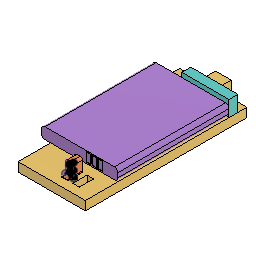
BatteryHolder (Autodesk Fusion 360 design; units mm, degrees)
Autodesk Fusion 360 part; units mm, degrees
sketch "Base" plane through (0, 0, 0) normal (0, 0, 1) x (1, 0, 0) in component "Rail"
  line L0 (0, 0) -> (30, 0)
  line L1 (30, 0) -> (30, 72)
  line L2 (30, 72) -> (0, 72)
  line L3 (0, 72) -> (0, 0)
  line L4 (21, 68) -> (18, 68)
  line L5 (18, 68) -> (18, 28)
  line L6 (18, 28) -> (21, 28)
  line L7 (21, 28) -> (21, 68)
  dimension "d1" = 30
  dimension "d2" = 72
  dimension "d45" = 3
  dimension "d46" = 9
  dimension "d47" = 40
  dimension "d48" = 4
  constraint horizontal L0
  constraint vertical L1
  constraint horizontal L2
  constraint vertical L3
  constraint coincident L0.start L3.end
  constraint horizontal L4
  constraint vertical L5
  constraint horizontal L6
  constraint vertical L7
  measures "d1" distance of L0.start L0.end
  measures "d2" distance of L0.start L2.end
  measures "d45" distance of L4.start L4.end
  measures "d46" distance of L1 L7
  measures "d47" distance of L4.start L6.end
  measures "d48" distance of L2 L4
extrude "Extrude1" add sketch "Base" along normal blind 4 makes body 1 in component "Rail"
sketch "BoltHolder" plane through (0, 0, 4) normal (0, 0, 1) x (-1, 0, 0) in component "Rail"
  line L0 (0, -72) -> (0, 0)
  line L1 (0, 0) -> (-30, 0)
  line L2 (-30, 0) -> (-30, -72)
  line L3 (-30, -72) -> (0, -72)
  line L4 (-23, -72) -> (-16, -72)
  line L5 (-16, -72) -> (-16, -68)
  line L6 (-16, -68) -> (-23, -68)
  line L7 (-23, -68) -> (-23, -72)
  line L8 (-30, 0) -> (-30, -72)
  line L9 (-21, -68) -> (-21, -28)
  line L10 (-21, -28) -> (-18, -28)
  line L11 (-18, -28) -> (-18, -68)
  line L12 (-18, -68) -> (-21, -68)
  dimension "d5" = 7
  dimension "d6" = 4
  dimension "d7" = 7
  constraint horizontal L4
  constraint vertical L5
  constraint horizontal L6
  constraint vertical L7
  constraint coincident L3 L4.start
  measures "d5" distance of L4.start L4.end
  measures "d6" distance of L4.start L6.end
  measures "d7" distance of L7 L8
extrude "Extrude3" add sketch "BoltHolder" along normal blind 7 contours L3 L4 L5 L6 L7 L12 bodies 1 in component "Rail"
sketch "BoltHole" plane through (0, 72, 0) normal (0, 1, 0) x (-1, 0, 0) in component "Rail"
  line L0 (-30, 0) -> (0, 0)
  line L1 (0, 0) -> (0, 4)
  line L2 (0, 4) -> (-16, 4)
  line L3 (-16, 4) -> (-16, 11)
  line L4 (-16, 11) -> (-23, 11)
  line L5 (-23, 11) -> (-23, 4)
  line L6 (-23, 4) -> (-30, 4)
  line L7 (-30, 4) -> (-30, 0)
  line L8 (-23, 11) -> (-16, 4) construction
  line L9 (-23, 4) -> (-16, 11) construction
  circle A0 centre (-19.5, 7.5) radius 1.25
  circle A1 centre (-19.5, 7.5) radius 2.5
  dimension "d12" = 2.5
  dimension "d13" = 5
  constraint coincident L4.end L5.start
  constraint coincident L2.end L3.start
  constraint coincident L5.end L6.start
  constraint coincident L3.end L4.start
  constraint midpoint L8 A0.centre
  constraint concentric A0 A1
  measures "d12" diameter of A0
  measures "d13" diameter of A1
extrude "Extrude4" cut sketch "BoltHole" against normal up to surface (4 mm away) contours A0 bodies 1 in component "Rail"
extrude "Extrude5" cut sketch "BoltHole" against normal blind 2 contours A1 bodies 1 in component "Rail"
sketch "Sketch1" plane through (0, 68, 0) normal (0, -1, 0) x (1, 0, 0) in component "Pusher"
  circle A0 centre (19.5, 7.5) radius 1.25
  line L0 (21, 4) -> (23, 4)
  line L1 (23, 4) -> (23, 11)
  line L2 (23, 11) -> (16, 11)
  line L3 (16, 11) -> (16, 4)
  line L4 (23, 11) -> (30, 11)
  line L5 (30, 11) -> (30, 4)
  line L6 (30, 4) -> (23, 4)
  line L7 (23, 4) -> (23, 11)
  line L8 (16, 11) -> (9, 11)
  line L9 (9, 11) -> (9, 4)
  line L10 (9, 4) -> (16, 4)
  line L11 (16, 4) -> (16, 11)
  line L12 (18, 0) -> (21, 0)
  line L13 (21, 0) -> (21, 4)
  line L14 (16, 4) -> (18, 4)
  line L15 (18, 4) -> (18, 0)
  point P0 (30, 4)
  dimension "d18" = 7
  constraint horizontal L4
  constraint vertical L5
  constraint horizontal L6
  constraint vertical L7
  constraint coincident P0 L5.end
  constraint coincident L1.end L2.start
  constraint horizontal L8
  constraint vertical L9
  constraint horizontal L10
  constraint vertical L11
  constraint coincident L2.end L3.start
  measures "d18" distance of L2.end L8.end
extrude "Extrude1'" add sketch "Sketch1" along normal blind 4 separate body contours A0 | L0 L1 L2 L3 L7 L11 L12 L13 L14 L15 | L1 L4 L5 L6 L7 | L3 L8 L9 L10 L11 makes body 2 in component "Pusher"
sketch "Sketch2" plane through (0, 68, 0) normal (0, 1, 0) x (-1, 0, 0) in component "Pusher"
  line L0 (-9, 11) -> (-30, 11)
  line L1 (-30, 11) -> (-30, 4)
  line L2 (-30, 4) -> (-21, 4)
  line L3 (-9, 4) -> (-9, 11)
  circle A0 centre (-19.5, 7.5) radius 1.25
  line L4 (-21, 4) -> (-21, 0)
  line L5 (-21, 0) -> (-18, 0)
  line L6 (-18, 0) -> (-18, 4)
  line L7 (-18, 4) -> (-9, 4)
extrude "Extrude2" cut sketch "Sketch2" against normal blind 2 contours A0 bodies 2 in component "Pusher"
sketch "Sketch1 (2)" plane through (0, 0, 4) normal (0, 0, 1) x (-1, 0, 0) in component "Connector"
  line L0 (-24.5, -4) -> (-14.5, -4)
  line L1 (-14.5, -4) -> (-14.5, -10)
  line L2 (-14.5, -10) -> (-24.5, -10)
  line L3 (-24.5, -10) -> (-24.5, -4)
  line L4 (0, 0) -> (-30, 0)
  line L5 (-19.5, -72) -> (-19.5, 0) construction
  point P0 (-19.5, -72)
  point P1 (-19.5, -4)
  dimension "d23" = 10
  dimension "d24" = 6
  dimension "d25" = 4
  constraint horizontal L0
  constraint vertical L1
  constraint horizontal L2
  constraint vertical L3
  constraint coincident P0 L5.start
  constraint coincident L4 L5.end
  constraint perpendicular L4 L5
  constraint coincident L5 P1
  constraint midpoint L0 P1
  measures "d23" distance of L0.start L0.end
  measures "d24" distance of L0.start L2.end
  measures "d25" distance of L5.end P1
extrude "Extrude1''" add sketch "Sketch1 (2)" along normal blind 6 separate body makes body 3 in component "Connector"
sketch "Sketch2 (2)" plane through (0, 10, 0) normal (0, 1, 0) x (-1, 0, 0) in component "Connector"
  line L0 (-24.5, 4) -> (-14.5, 4)
  line L1 (-14.5, 4) -> (-14.5, 10)
  line L2 (-14.5, 10) -> (-24.5, 10)
  line L3 (-24.5, 10) -> (-24.5, 4)
  line L4 (-24.5, 10) -> (-14.5, 4) construction
  line L5 (-24.5, 4) -> (-14.5, 10) construction
  circle A0 centre (-19.5, 7) radius 0.75
  dimension "d28" = 1.5
  constraint coincident L2.end L3.start
  constraint coincident L0.end L1.start
  constraint coincident L0.start L3.end
  constraint coincident L1.end L2.start
  constraint midpoint L4 A0.centre
  measures "d28" diameter of A0
extrude "Extrude2'" cut sketch "Sketch2 (2)" against normal up to surface (6 mm away) contours A0 bodies 3 in component "Connector"
pattern_linear "R-Pattern1" count 3 spacing 2.5 along (1, 0, 0) both ways of "Extrude2'" in component "Connector"
sketch "Sketch3" plane through (0, 10, 0) normal (0, 1, 0) x (-1, 0, 0) in component "Connector"
  circle A0 centre (-22, 7) radius 0.75
  line L0 (-24.5, 4) -> (-14.5, 4)
  line L1 (-14.5, 4) -> (-14.5, 10)
  line L2 (-14.5, 10) -> (-24.5, 10)
  line L3 (-24.5, 10) -> (-24.5, 4)
  line L4 (-24.5, 10) -> (-14.5, 4) construction
  line L5 (-24.5, 4) -> (-14.5, 10) construction
  line L6 (-15.3, 5.75) -> (-23.7, 5.75)
  line L7 (-23.7, 5.75) -> (-23.7, 8.25)
  line L8 (-23.7, 8.25) -> (-15.3, 8.25)
  line L9 (-15.3, 8.25) -> (-15.3, 5.75)
  circle A1 centre (-17, 7) radius 0.75
  circle A2 centre (-19.5, 7) radius 0.75
  point P0 (-19.5, 7)
  dimension "d35" = 8.4
  dimension "d36" = 2.5
  constraint coincident L2.end L3.start
  constraint coincident L0.end L1.start
  constraint coincident L0.start L3.end
  constraint coincident L1.end L2.start
  constraint horizontal L6
  constraint perpendicular L6 L7
  constraint parallel L6 L8
  constraint parallel L7 L9
  measures "d35" distance of L7.end L8.end
  measures "d36" distance of L6.end L7.end
extrude "Extrude3'" cut sketch "Sketch3" against normal blind 5.5 contours L6 L7 L8 L9 | A1 | A2 bodies 3 in component "Connector"
sketch "Sketch4" plane through (0, 0, 4) normal (0, 0, -1) x (1, 0, 0) in component "Connector"
  line L0 (14.5, -10) -> (24.5, -10)
  line L1 (24.5, -10) -> (24.5, -4)
  line L2 (24.5, -4) -> (14.5, -4)
  line L3 (14.5, -4) -> (14.5, -10)
  line L4 (19.5, -4) -> (19.5, -10) construction
  line L5 (15.75, -4) -> (18.25, -4)
  line L6 (18.25, -4) -> (18.25, -10)
  line L7 (18.25, -10) -> (15.75, -10)
  line L8 (15.75, -10) -> (15.75, -4)
  line L9 (23.25, -10) -> (23.25, -4)
  line L10 (23.25, -4) -> (20.75, -4)
  line L11 (20.75, -10) -> (23.25, -10)
  line L12 (20.75, -4) -> (20.75, -10)
  line L13 (18.75, -4) -> (20.25, -4)
  line L14 (16.25, -4) -> (17.75, -4)
  point P0 (17, -4)
  dimension "d39" = 2.5
  constraint midpoint L2 L4.start
  constraint midpoint L0 L4.end
  constraint horizontal L5
  constraint vertical L6
  constraint horizontal L7
  constraint vertical L8
  constraint coincident L2 L5.start
  constraint midpoint L5 P0
  constraint symmetric L4 L5.start L9.end
  constraint symmetric L4 L5.end L10.end
  constraint symmetric L4 L6.end L11.start
  constraint symmetric L4 L7.end L9.start
  measures "d39" distance of L5.start L5.end
extrude "Extrude4'" add sketch "Sketch4" along normal blind 4 contours L0 L2 L5 L6 L7 L8 L14 | L0 L2 L9 L10 L11 L12 bodies 3 in component "Connector"
sketch "CutoutConnector" plane through (0, 0, 0) normal (0, 0, 1) x (1, 0, 0) in component "Rail"
  line L0 (15.75, 4) -> (18.25, 4)
  line L1 (18.25, 4) -> (18.25, 10)
  line L2 (18.25, 10) -> (15.75, 10)
  line L3 (15.75, 10) -> (15.75, 4)
  line L4 (20.75, 4) -> (23.25, 4)
  line L5 (23.25, 4) -> (23.25, 10)
  line L6 (23.25, 10) -> (20.75, 10)
  line L7 (20.75, 10) -> (20.75, 4)
  line L8 (18.45, 3.8) -> (18.45, 10.2)
  line L9 (18.45, 10.2) -> (15.55, 10.2)
  line L10 (15.55, 10.2) -> (15.55, 3.8)
  line L11 (15.55, 3.8) -> (18.45, 3.8)
  line L12 (20.55, 10.2) -> (20.55, 3.8)
  line L13 (20.55, 3.8) -> (23.45, 3.8)
  line L14 (23.45, 3.8) -> (23.45, 10.2)
  line L15 (23.45, 10.2) -> (20.55, 10.2)
  point P0 (15.75, 4)
  point P1 (18.25, 10)
  point P2 (20.75, 4)
  point P3 (23.25, 10)
  dimension "d42" = 0.2
  constraint horizontal L0
  constraint vertical L1
  constraint horizontal L2
  constraint vertical L3
  constraint coincident P1 L1.end
  constraint coincident P0 L0.start
  constraint horizontal L4
  constraint vertical L5
  constraint horizontal L6
  constraint vertical L7
  constraint coincident P3 L5.end
  constraint coincident P2 L4.start
extrude "Extrude6" cut sketch "CutoutConnector" along normal up to surface (4 mm away) contours L0 L1 L2 L3 | L4 L5 L6 L7 | L8 L9 L10 L11 | L12 L13 L14 L15 bodies 1 in component "Rail"
sketch "Sketch1 (3)" plane through (0, 0, 4) normal (0, 0, 1) x (-1, 0, 0) in component "WireConnector"
  line L0 (-18.45, -10.2) -> (-18.45, -3.8)
  line L1 (-18.45, -3.8) -> (-15.55, -3.8)
  line L2 (-15.55, -3.8) -> (-15.55, -10.2)
  line L3 (-15.55, -10.2) -> (-18.45, -10.2)
  line L4 (-16, -68) -> (-16, -72)
  line L5 (-16, -72) -> (0, -72)
  line L6 (0, -72) -> (0, 0)
  line L7 (0, 0) -> (-30, 0)
  line L8 (-30, 0) -> (-30, -72)
  line L9 (-30, -72) -> (-23, -72)
  line L10 (-23, -72) -> (-23, -68)
  line L11 (-23, -68) -> (-21, -68)
  line L12 (-21, -68) -> (-21, -28)
  line L13 (-21, -28) -> (-18, -28)
  line L14 (-18, -28) -> (-18, -68)
  line L15 (-18, -68) -> (-16, -68)
  line L16 (-15.55, -10.2) -> (-18.45, -10.2)
  line L17 (-18.45, -10.2) -> (-18.45, -3.8)
  line L18 (-18.45, -3.8) -> (-15.55, -3.8)
  line L19 (-15.55, -3.8) -> (-15.55, -10.2)
  line L20 (-18.25, -10) -> (-18.25, -4)
  line L21 (-18.25, -4) -> (-15.75, -4)
  line L22 (-15.75, -4) -> (-15.75, -10)
  line L23 (-15.75, -10) -> (-18.25, -10)
  constraint horizontal L16
  constraint vertical L17
  constraint horizontal L18
  constraint vertical L19
  constraint coincident L0.end L1.start
  constraint coincident L2.end L3.start
  constraint parallel L17 L20
  constraint parallel L18 L21
  constraint parallel L19 L22
  constraint parallel L16 L23
extrude "Extrude1'''" add sketch "Sketch1 (3)" against normal up to surface (4 mm away) separate body contours L20 L21 L22 L23 makes body 4 in component "WireConnector"
sketch "Sketch2 (3)" plane through (0, 0, 4) normal (0, 0, 1) x (-1, 0, 0) in component "WireConnector"
  line L0 (-15.75, -10) -> (-15.75, -4)
  line L1 (-15.75, -4) -> (-18.25, -4)
  line L2 (-18.25, -4) -> (-18.25, -10)
  line L3 (-18.25, -10) -> (-15.75, -10)
  line L4 (-15.75, -10) -> (-18.25, -10)
  line L5 (-18.25, -10) -> (-18.25, -6)
  line L6 (-18.25, -6) -> (-15.75, -6)
  line L7 (-15.75, -6) -> (-15.75, -10)
  line L8 (-18.25, -10) -> (-18.75, -10)
  line L9 (-18.75, -10) -> (-18.75, -6)
  line L10 (-18.75, -6) -> (-18.25, -6)
  line L11 (-18.25, -6) -> (-18.25, -10)
  line L12 (-15.75, -10) -> (-15.25, -10)
  line L13 (-15.25, -10) -> (-15.25, -6)
  line L14 (-15.25, -6) -> (-15.75, -6)
  line L15 (-15.75, -6) -> (-15.75, -10)
  dimension "d52" = 4
  dimension "d94" = 0.5
  dimension "d95" = 4
  dimension "d96" = 0.5
  constraint horizontal L4
  constraint vertical L5
  constraint horizontal L6
  constraint vertical L7
  constraint coincident L0.start L3.end
  constraint horizontal L8
  constraint vertical L9
  constraint horizontal L10
  constraint vertical L11
  constraint coincident L2.end L3.start
  constraint horizontal L12
  constraint vertical L13
  constraint horizontal L14
  constraint vertical L15
  measures "d52" distance of L0.start L6.end
  measures "d94" distance of L2.end L8.end
  measures "d95" distance of L2.end L5.end
  measures "d96" distance of L0.start L12.end
extrude "Extrude2''" add sketch "Sketch2 (3)" along normal blind 6 contours L0 L2 L3 L4 L5 L6 L7 L11 L15 | L0 L7 L12 L13 L14 L15 | L2 L5 L8 L9 L10 L11 bodies 4 in component "WireConnector"
sketch "Sketch3 (2)" plane through (0, 6, 0) normal (0, -1, 0) x (1, 0, 0) in component "WireConnector"
  line L0 (15.75, 4) -> (18.75, 4)
  line L1 (18.75, 10) -> (15.25, 10)
  line L2 (17.5, 4) -> (18.549, 4) construction
  line L3 (17.5, 4) -> (18.25, 4) construction
  line L4 (18.75, 7) -> (15.25, 7) construction
  line L5 (18.75, 10) -> (15.25, 7) construction
  line L6 (15.25, 7) -> (18.75, 4) construction
  circle A0 centre (17, 8.5) radius 0.75
  circle A1 centre (17, 5.5) radius 1
  circle A2 centre (17, 8.5) radius 1
  line L7 (15.25, 4) -> (15.75, 4)
  line L8 (18.25, 4) -> (18.75, 4)
  line L9 (18.75, 4) -> (18.75, 10)
  line L10 (15.25, 10) -> (15.25, 4)
  dimension "d66" = 1.5
  dimension "d67" = 2
  dimension "d88" = 2
  constraint horizontal L2
  constraint coincident L3.end L8.start
  constraint coincident L1.start L5.start
  constraint midpoint L5 A0.centre
  constraint midpoint L6 A1.centre
  constraint concentric A0 A2
  constraint coincident L0.end L6.end
  constraint midpoint L4.end L10
  constraint coincident L4.start L9
  constraint midpoint L4.start L9
  measures "d66" diameter of A0
  measures "d67" diameter of A1
  measures "d88" diameter of A2
extrude "Extrude4''" cut sketch "Sketch3 (2)" against normal up to surface (4 mm away) contours A0 | A1 bodies 4 in component "WireConnector"
sketch "Sketch1 (4)" plane through (0, 64, 0) normal (0, -1, 0) x (1, 0, 0) in component "Battery"
  line L0 (30, 11) -> (9, 11)
  line L1 (9, 11) -> (9, 4)
  line L2 (9, 4) -> (18, 4)
  line L3 (18, 4) -> (18, 0)
  line L4 (18, 0) -> (21, 0)
  line L5 (21, 0) -> (21, 4)
  line L6 (21, 4) -> (30, 4)
  line L7 (30, 4) -> (30, 11)
  line L8 (30, 4) -> (-4, 4)
  line L9 (-4, 4) -> (-4, 9)
  line L10 (-4, 9) -> (30, 9)
  line L11 (30, 9) -> (30, 4)
  dimension "d68" = 34
  dimension "d69" = 5
  constraint horizontal L8
  constraint vertical L9
  constraint horizontal L10
  constraint vertical L11
  constraint coincident L6.end L7.start
  measures "d68" distance of L6.end L8.end
  measures "d69" distance of L6.end L10.end
extrude "Extrude1''''" add sketch "Sketch1 (4)" along normal blind 49.5 separate body contours L1 L2 L6 L7 L8 L10 L11 | L1 L8 L9 L10 makes body 5 in component "Battery"
sketch "Sketch2 (4)" plane through (0, 14.5, 0) normal (0, -1, 0) x (1, 0, 0) in component "Battery"
  line L0 (30, 9) -> (-4, 9)
  line L1 (-4, 9) -> (-4, 4)
  line L2 (-4, 4) -> (30, 4)
  line L3 (30, 4) -> (30, 9)
  line L4 (23, 8.5) -> (21, 8.5)
  line L5 (21, 8.5) -> (21, 4.5)
  line L6 (21, 4.5) -> (23, 4.5)
  line L7 (23, 4.5) -> (23, 8.5)
  dimension "d78" = 7
  dimension "d79" = 0.5
  dimension "d80" = 0.5
  dimension "d81" = 2
  constraint horizontal L4
  constraint vertical L5
  constraint horizontal L6
  constraint vertical L7
  measures "d78" distance of L3 L7
  measures "d79" distance of L0 L4
  measures "d80" distance of L2 L6
  measures "d81" distance of L4.start L4.end
extrude "Extrude2'''" cut sketch "Sketch2 (4)" against normal blind 0.2 contours L4 L5 L6 L7 bodies 5 in component "Battery"
pattern_linear "R-Pattern1'" count 3 spacing 2.5 along (-1, 0, 0) of "Extrude2'''" in component "Battery"
extrude "Extrude5'" cut sketch "Sketch3 (2)" against normal blind 2.5 contours A2 bodies 4 in component "WireConnector"
fillet "Fillet2" radius 1 4 edges at (18.75, 8, 10) (15.25, 8, 10) (15.25, 8, 4) (18.75, 8, 4) on bodies 4 in component "WireConnector"
fillet "Fillet1" radius 1.5 4 edges at (30, 39.25, 9) (30, 39.25, 4) (-4, 39.25, 4) (-4, 39.25, 9) on bodies 5 in component "Battery"
extrude "Extrude2''''" [suppressed] in component "Rail"
component "Rail" placed x (1, 0, 0) y (0, 1, 0) z (0, 0, 1) at (0, 0, 0)
component "Pusher" placed x (1, 0, 0) y (0, 1, 0) z (0, 0, 1) at (0, 0, 0)
component "Connector" placed x (1, 0, 0) y (0, 1, 0) z (0, 0, 1) at (0, 0, 0)
component "WireConnector" placed x (1, 0, 0) y (0, 1, 0) z (0, 0, 1) at (0, 0, 0)
component "Battery" placed x (1, 0, 0) y (0, 1, 0) z (0, 0, 1) at (0, 0, 0)
named bodies: "Rail"
